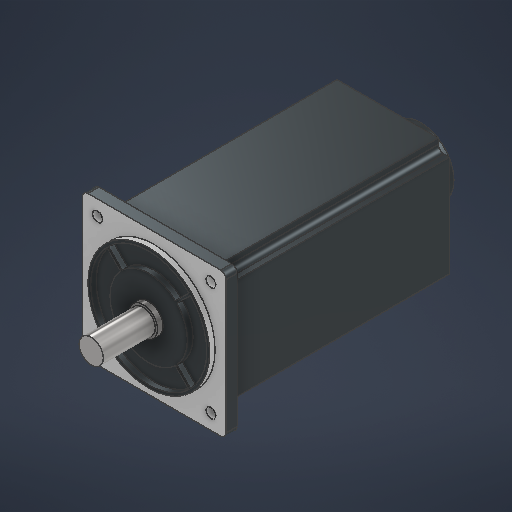
# Autodesk Inventor part: SERVOMOTOR-2.3KWv1
Saved by Autodesk Inventor 2025.3 (Build 293356030, 356C)
## iProperties
Created: 2025-10-05
Part Number: SERVOMOTOR-2.3KWv1
Material: Generic
Document SubType Name: Modeling
Designer: lstk1ng
Density: 1 g/cm^3
Appearance: Default
Author: lstk1ng
Autodesk Inventor part; units mm, degrees
ref_plane "YZ Plane" through (0, 0, 0) normal (1, 0, 0) x (0, 1, 0)
ref_plane "XZ Plane" through (0, 0, 0) normal (0, 1, 0) x (-1, 0, 0)
ref_plane "XY Plane" through (0, 0, 0) normal (0, 0, 1) x (1, 0, 0)
sketch "Sketch1" plane through (0, 0, 0) normal (0, 0, 1) x (1, 0, 0)
  line L0 (65, -65) -> (-65, -65)
  line L1 (-65, -65) -> (-65, 65)
  line L2 (-65, 65) -> (65, 65)
  line L3 (65, 65) -> (65, -65)
  line L4 (65, -65) -> (-65, 65) construction
  line L5 (-65, -65) -> (65, 65) construction
  circle A0 centre (0, 0) radius 72.5 construction
  circle A1 centre (-51.2652, 51.2652) radius 4.5
  circle A2 centre (51.2652, 51.2652) radius 4.5
  line L6 (-65, 0) -> (65, 0) construction
  circle A3 centre (-51.2652, -51.2652) radius 4.5
  circle A4 centre (51.2652, -51.2652) radius 4.5
  dimension "d0" = 130
  dimension "d1" = 130
  dimension "d2" = 145
  dimension "d3" = 9
  dimension "d4" = 9
  constraints: 14 end point, 5 centre point, 4 midpoint, 2 parallel, 2 point on circle, 2 point on line, 2 symmetric about line, 1 coincident, 1 horizontal, 1 perpendicular, 2 other
  measures "d0" distance of L1.end L2.end
  measures "d1" distance of L0.end L1.end
  measures "d2" diameter of A0
  measures "d3" diameter of A1
  measures "d4" diameter of A2
extrude "Extrusion1" add sketch "Sketch1" along normal blind 10
fillet "Fillet1" radius 5 4 edges at (-65, -65, 5) (65, -65, 5) (65, 65, 5) (-65, 65, 5)
sketch "Sketch2" plane through (0, 0, 10) normal (0, 0, 1) x (1, 0, 0)
  circle A0 centre (0, 0) radius 55
  circle A1 centre (0, 0) radius 54
  dimension "d8" = 110
  constraints: 2 centre point, 1 coincident
  measures "d8" diameter of A0
extrude "Extrusion2" add sketch "Sketch2" along normal blind 5
sketch "Sketch3" plane through (0, 0, 10) normal (0, 0, 1) x (1, 0, 0)
  circle A0 centre (0, 0) radius 15
  line L0 (0, 0) -> (24.7487, -24.7487) construction
  line L1 (0, 0) -> (35, 0) construction
  line L2 (0, 0) -> (-24.7487, -24.7487) construction
  line L3 (0, 0) -> (35, 0) construction
  line L4 (0, 0) -> (24.7487, 24.7487) construction
  line L5 (0, 0) -> (-24.7487, 24.7487) construction
  line L6 (0.7071, 0.7071) -> (-24.0416, 25.4558) construction
  line L7 (37.8235, -36.4093) -> (25.4457, -24.0315)
  line L8 (36.4093, -37.8235) -> (24.0315, -25.4457)
  line L9 (-36.4093, -37.8235) -> (-24.0315, -25.4457)
  line L10 (-37.8235, -36.4093) -> (-25.4457, -24.0315)
  line L11 (-25.4457, 24.0315) -> (-37.8235, 36.4093)
  line L12 (-24.0315, 25.4457) -> (-36.4093, 37.8235)
  line L13 (-25.4457, 24.0315) -> (-25.4558, 24.0416)
  line L14 (-24.0315, 25.4457) -> (-24.0416, 25.4558)
  line L15 (-25.4457, 24.0315) -> (-25.4558, 24.0416)
  line L16 (36.4093, 37.8235) -> (24.0315, 25.4457)
  line L17 (37.8235, 36.4093) -> (25.4457, 24.0315)
  arc A1 (-24.0315, -25.4457) -> (24.0315, -25.4457) centre (0, 0) ccw
  arc A2 (-25.4457, 24.0315) -> (-25.4457, -24.0315) centre (0, 0) ccw
  arc A3 (25.4457, -24.0315) -> (25.4457, 24.0315) centre (0, 0) ccw
  arc A4 (24.0315, 25.4457) -> (-24.0315, 25.4457) centre (0, 0) ccw
  arc A5 (-36.4093, -37.8235) -> (36.4093, -37.8235) centre (0, 0) ccw
  arc A6 (-37.8235, 36.4093) -> (-37.8235, -36.4093) centre (0, 0) ccw
  arc A7 (37.8235, -36.4093) -> (37.8235, 36.4093) centre (0, 0) ccw
  arc A8 (36.4093, 37.8235) -> (-36.4093, 37.8235) centre (0, 0) ccw
  circle A9 centre (0, 0) radius 54 projected
  dimension "d12" = 30
  dimension "d14" = 45
  dimension "d15" = 135
  constraints: 36 end point, 17 point on circle, 9 centre point, 2 equal length, 2 horizontal, 2 symmetric about line, 1 coincident, 1 point on line
  measures "d12" diameter of A0
  measures "d14" angle of L0 L1
  measures "d15" angle of L2 L3
extrude "Extrusion3" add sketch "Sketch3" along normal blind 5
sketch "Sketch4" plane through (0, 0, 0) normal (0, 1, 0) x (-1, 0, 0)
  line L0 (15, 15) -> (15, 10) projected
  line L1 (15, 10) -> (15, 15)
  line L2 (0, 15) -> (11, 15) construction
  line L3 (15, 15) -> (13, 15)
  line L4 (13, 15) -> (13, 20)
  line L5 (11, 16) -> (11, 67) construction
  line L6 (60, 10) -> (65, 10) construction
  line L7 (13, 20) -> (11, 20)
  line L8 (11, 67) -> (11, 20)
  line L9 (11, 67) -> (0, 67)
  line L10 (0, 67) -> (0, 10)
  line L11 (15, 10) -> (0, 10)
  line L12 (0, -13.4) -> (0, 80.4) projected
  point P0 (0, 0)
  dimension "d18" = 11
  dimension "d19" = 2
  dimension "d20" = 5
  dimension "d21" = 57
  constraints: 20 end point, 3 point on line, 2 perpendicular, 2 vertical, 1 horizontal
  measures "d18" distance of L2.start L2.end
  measures "d19" distance of L1.end L3.end
  measures "d20" distance of L3.end L4.end
  measures "d21" distance from line of L6 L5.end
revolve "Revolution1" add sketch "Sketch4" angle 360 about axis through (0, 0, -10) along (0, 0, 1)
sketch "Sketch5" plane through (0, 0, 0) normal (0, 0, -1) x (-1, 0, 0)
  line L0 (-45.7652, 55.7652) -> (45.7652, 55.7652)
  line L1 (55.7652, 45.7652) -> (55.7652, -45.7652)
  line L2 (45.7652, -55.7652) -> (-45.7652, -55.7652)
  line L3 (-55.7652, -45.7652) -> (-55.7652, 45.7652)
  line L4 (-55.7652, 55.7652) -> (55.7652, -55.7652) construction
  line L5 (55.7652, 55.7652) -> (-55.7652, -55.7652) construction
  line L6 (55.7652, -55.7652) -> (55.7652, -45.7652) construction
  line L7 (55.7652, -45.7652) -> (50.7652, -45.7652)
  line L8 (45.7652, -55.7652) -> (45.7652, -50.7652)
  arc A0 (50.7652, -45.7652) -> (45.7652, -50.7652) centre (50.7652, -50.7652) ccw
  line L9 (0, 0) -> (0, -55.7652) construction
  line L10 (0, 0) -> (-55.7652, 0) construction
  line L11 (-55.7652, -45.7652) -> (-50.7652, -45.7652)
  line L12 (-45.7652, -55.7652) -> (-45.7652, -50.7652)
  arc A1 (-45.7652, -50.7652) -> (-50.7652, -45.7652) centre (-50.7652, -50.7652) ccw
  line L13 (55.7652, 45.7652) -> (50.7652, 45.7652)
  line L14 (45.7652, 55.7652) -> (45.7652, 50.7652)
  arc A2 (45.7652, 50.7652) -> (50.7652, 45.7652) centre (50.7652, 50.7652) ccw
  line L15 (-45.7652, 55.7652) -> (-45.7652, 50.7652)
  arc A3 (-50.7652, 45.7652) -> (-45.7652, 50.7652) centre (-50.7652, 50.7652) ccw
  line L16 (-55.7652, 45.7652) -> (-50.7652, 45.7652)
  point P0 (45.7652, -45.7652)
  dimension "d23" = 10
  dimension "d24" = 5
  constraints: 34 end point, 15 symmetric about line, 8 point on circle, 4 centre point, 4 midpoint, 4 perpendicular, 3 point on line, 2 parallel, 2 tangent, 1 horizontal, 3 other
  measures "d23" distance of L1.end L4.end
  measures "d24" radius of A0
extrude "Extrusion4" add sketch "Sketch5" along normal blind 201
sketch "Sketch6" plane through (0, 0, -201) normal (0, 0, -1) x (-1, 0, 0)
  circle A0 centre (0, 0) radius 30
  dimension "d27" = 60
  constraints: 1 centre point, 1 coincident
  measures "d27" diameter of A0
extrude "Extrusion5" add sketch "Sketch6" along normal blind 30
body "Solid1"
